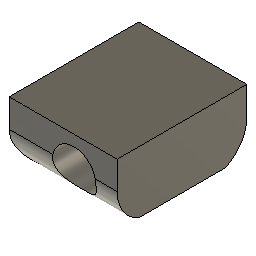
tof_switch (Autodesk Fusion 360 design; units mm, degrees)
Autodesk Fusion 360 part; units mm, degrees
sketch "Sketch1" plane through (0, 0, 0) normal (0, 0, 1) x (1, 0, 0)
  line L0 (-25, 25) -> (25, 25)
  line L1 (25, 25) -> (25, -25)
  line L2 (25, -25) -> (-25, -25)
  line L3 (-25, -25) -> (-25, 25)
  constraint horizontal L0
  constraint vertical L1
  constraint horizontal L2
  constraint vertical L3
extrude "Extrude1" add sketch "Sketch1" along normal blind 25
sketch "Sketch2" plane through (0, -25, 0) normal (0, -1, 0) x (1, 0, 0)
  line L0 (-25, 0) -> (25, 0)
  line L1 (25, 0) -> (25, 25)
  line L2 (25, 25) -> (-25, 25)
  line L3 (-25, 25) -> (-25, 0)
  circle A0 centre (0, 25) radius 5
  dimension "d3" = 10
  constraint midpoint L2 A0.centre
  measures "d3" diameter of A0
extrude "Extrude2" cut sketch "Sketch2" against normal blind 66 contours L2 A0 | L2 A0
extrude "Extrude3" add 1 faces at (-18.3333, 8.3333, 25) along direction (0, 0, 1) blind 25
extrude "Extrude4" add 1 faces at (11.6667, -8.3333, 25) along direction (0, 0, 1) blind 25
extrude "Extrude5" add 1 faces at (-5, -8.3333, 41.6667) along direction (1, 0, 0) blind 10
sketch "Sketch4" plane through (0, -25, 0) normal (0, -1, 0) x (1, 0, 0)
  arc A0 (-5, 25) -> (5, 25) centre (0, 25) ccw
  line L0 (-5, 25) -> (5, 25)
  line L1 (25, 50) -> (-25, 50)
  line L2 (-25, 50) -> (-25, 0)
  line L3 (-25, 0) -> (25, 0)
  line L4 (25, 0) -> (25, 50)
  circle A1 centre (0, 25) radius 5
  dimension "d12" = 10
  constraint concentric A0 A1
  measures "d12" diameter of A1
extrude "Extrude6" cut sketch "Sketch4" against normal blind 105 contours L0 A1
extrude "Extrude7" cut 1 faces at (-8.3333, -8.3333, 50) along direction (0, 0, -1) blind 10
extrude "Extrude8" cut 1 faces at (-8.3333, 8.3333, 0) along direction (0, 0, 1) blind 10
extrude "Extrude9" cut 1 faces at (-8.3333, 8.3333, 10) along direction (0, 0, 1) blind 5
extrude "Extrude10" cut 1 faces at (-8.3333, -8.3333, 40) along direction (0, 0, -1) blind 7
extrude "Extrude11" cut 1 faces at (-8.3333, 8.3333, 15) along direction (0, 0, 1) blind 2
extrude "Extrude12" cut 1 faces at (25, 8.3333, 22.3333) along direction (-1, 0, 0) blind 10
extrude "Extrude13" cut 1 faces at (-25, -8.3333, 22.3333) along direction (1, 0, 0) blind 10
extrude "Extrude14" cut 1 faces at (11.6667, 25, 25) along direction (0, -1, 0) blind 20
extrude "Extrude15" cut 1 faces at (-5, -15, 33) along direction (0, 0, -1) blind 0.5
extrude "Extrude16" cut 1 faces at (-5, -5, 17) along direction (0, 0, 1) blind 0.5
fillet "Fillet1" radius 8.5 1 faces at (-5, -5, 17.5)
thread "Thread4" "ACME Screw Threads 3/8 0.3750 0.3750 4G" major diameter 9.906 minor diameter 7.4727 pitch 2.1167 angle 29 resizes the face on face at (3.7262, -5, 28.334)
extrude "Extrude17" cut 1 faces at (15, -5, 28.1667) along direction (-1, 0, 0) blind 5
extrude "Extrude18" cut 1 faces at (13.3333, -5, 26) along direction (0, 0, -1) blind 10
sketch "Sketch7" plane through (0, -25, 0) normal (0, -1, 0) x (1, 0, 0)
  line L0 (10, 26) -> (10, 32.5)
  line L1 (10, 32.5) -> (-15, 32.5)
  line L2 (-15, 32.5) -> (-15, 26)
  line L3 (-15, 26) -> (-3.6, 26)
  arc A0 (3.6, 26) -> (-3.6, 26) centre (0, 25) ccw
  line L4 (3.6, 26) -> (10, 26)
  circle A1 centre (0, 25) radius 5
  dimension "d51" = 10
  constraint concentric A0 A1
  measures "d51" diameter of A1
extrude "Extrude19" cut sketch "Sketch7" against normal blind 42 contours L3 A0 L4 A1 | L3 A0 L4 A1
